Autodesk Fusion 360 part; units mm, degrees
(part 2 of 2)
  arc A307 (-22.8615, 180.477) -> (-23.3615, 180.977) centre (-23.3615, 180.477) ccw
  line L308 (-36.8615, 186.527) -> (-36.8615, 199.527)
  line L309 (-22.8615, 186.527) -> (-22.8615, 199.527)
  line L310 (-36.3615, 186.027) -> (-23.3615, 186.027)
  line L311 (-36.3615, 200.027) -> (-23.3615, 200.027)
  arc A308 (-36.8615, 186.527) -> (-36.3615, 186.027) centre (-36.3615, 186.527) ccw
  arc A309 (-36.3615, 200.027) -> (-36.8615, 199.527) centre (-36.3615, 199.527) ccw
  arc A310 (-23.3615, 186.027) -> (-22.8615, 186.527) centre (-23.3615, 186.527) ccw
  arc A311 (-22.8615, 199.527) -> (-23.3615, 200.027) centre (-23.3615, 199.527) ccw
  line L312 (-36.8615, 205.577) -> (-36.8615, 218.577)
  line L313 (-22.8615, 205.577) -> (-22.8615, 218.577)
  line L314 (-36.3615, 205.077) -> (-23.3615, 205.077)
  line L315 (-36.3615, 219.077) -> (-23.3615, 219.077)
  arc A312 (-36.8615, 205.577) -> (-36.3615, 205.077) centre (-36.3615, 205.577) ccw
  arc A313 (-36.3615, 219.077) -> (-36.8615, 218.577) centre (-36.3615, 218.577) ccw
  arc A314 (-23.3615, 205.077) -> (-22.8615, 205.577) centre (-23.3615, 205.577) ccw
  arc A315 (-22.8615, 218.577) -> (-23.3615, 219.077) centre (-23.3615, 218.577) ccw
  line L316 (-36.8615, 224.627) -> (-36.8615, 237.627)
  line L317 (-22.8615, 224.627) -> (-22.8615, 237.627)
  line L318 (-36.3615, 224.127) -> (-23.3615, 224.127)
  line L319 (-36.3615, 238.127) -> (-23.3615, 238.127)
  arc A316 (-36.8615, 224.627) -> (-36.3615, 224.127) centre (-36.3615, 224.627) ccw
  arc A317 (-36.3615, 238.127) -> (-36.8615, 237.627) centre (-36.3615, 237.627) ccw
  arc A318 (-23.3615, 224.127) -> (-22.8615, 224.627) centre (-23.3615, 224.627) ccw
  arc A319 (-22.8615, 237.627) -> (-23.3615, 238.127) centre (-23.3615, 237.627) ccw
  line L320 (-36.8615, 260.3457) -> (-36.8615, 273.3457)
  line L321 (-22.8615, 260.3457) -> (-22.8615, 273.3457)
  line L322 (-36.3615, 259.8457) -> (-23.3615, 259.8457)
  line L323 (-36.3615, 273.8457) -> (-23.3615, 273.8457)
  arc A320 (-36.8615, 260.3457) -> (-36.3615, 259.8457) centre (-36.3615, 260.3457) ccw
  arc A321 (-36.3615, 273.8457) -> (-36.8615, 273.3457) centre (-36.3615, 273.3457) ccw
  arc A322 (-23.3615, 259.8457) -> (-22.8615, 260.3457) centre (-23.3615, 260.3457) ccw
  arc A323 (-22.8615, 273.3457) -> (-23.3615, 273.8457) centre (-23.3615, 273.3457) ccw
  line L324 (-35.8615, 251.9077) -> (-35.8615, 257.9077)
  line L325 (-20.8615, 251.9077) -> (-20.8615, 257.9077)
  line L326 (-35.3615, 251.4077) -> (-21.3615, 251.4077)
  line L327 (-35.3615, 258.4077) -> (-21.3615, 258.4077)
  arc A324 (-35.8615, 251.9077) -> (-35.3615, 251.4077) centre (-35.3615, 251.9077) ccw
  arc A325 (-35.3615, 258.4077) -> (-35.8615, 257.9077) centre (-35.3615, 257.9077) ccw
  arc A326 (-21.3615, 251.4077) -> (-20.8615, 251.9077) centre (-21.3615, 251.9077) ccw
  arc A327 (-20.8615, 257.9077) -> (-21.3615, 258.4077) centre (-21.3615, 257.9077) ccw
  line L328 (-35.8615, 275.7837) -> (-35.8615, 281.7837)
  line L329 (-20.8615, 275.7837) -> (-20.8615, 281.7837)
  line L330 (-35.3615, 275.2837) -> (-21.3615, 275.2837)
  line L331 (-35.3615, 282.2837) -> (-21.3615, 282.2837)
  arc A328 (-35.8615, 275.7837) -> (-35.3615, 275.2838) centre (-35.3615, 275.7837) ccw
  arc A329 (-35.3615, 282.2837) -> (-35.8615, 281.7837) centre (-35.3615, 281.7837) ccw
  arc A330 (-21.3615, 275.2837) -> (-20.8615, 275.7837) centre (-21.3615, 275.7837) ccw
  arc A331 (-20.8615, 281.7837) -> (-21.3615, 282.2837) centre (-21.3615, 281.7837) ccw
  line L332 (-36.8615, 319.877) -> (-36.8615, 332.877)
  line L333 (-22.8615, 319.877) -> (-22.8615, 332.877)
  line L334 (-36.3615, 319.377) -> (-23.3615, 319.377)
  line L335 (-36.3615, 333.377) -> (-23.3615, 333.377)
  arc A332 (-36.8615, 319.877) -> (-36.3615, 319.377) centre (-36.3615, 319.877) ccw
  arc A333 (-36.3615, 333.377) -> (-36.8615, 332.877) centre (-36.3615, 332.877) ccw
  arc A334 (-23.3615, 319.377) -> (-22.8615, 319.877) centre (-23.3615, 319.877) ccw
  arc A335 (-22.8615, 332.877) -> (-23.3615, 333.377) centre (-23.3615, 332.877) ccw
  line L336 (-17.8115, 12.6957) -> (-17.8115, 25.6957)
  line L337 (-3.8115, 12.6957) -> (-3.8115, 25.6957)
  line L338 (-17.3115, 12.1957) -> (-4.3115, 12.1957)
  line L339 (-17.3115, 26.1957) -> (-4.3115, 26.1957)
  arc A336 (-17.8115, 12.6957) -> (-17.3115, 12.1957) centre (-17.3115, 12.6957) ccw
  arc A337 (-17.3115, 26.1957) -> (-17.8115, 25.6957) centre (-17.3115, 25.6957) ccw
  arc A338 (-4.3115, 12.1957) -> (-3.8115, 12.6957) centre (-4.3115, 12.6957) ccw
  arc A339 (-3.8115, 25.6957) -> (-4.3115, 26.1957) centre (-4.3115, 25.6957) ccw
  line L340 (-17.8115, 36.5082) -> (-17.8115, 49.5082)
  line L341 (-3.8115, 36.5082) -> (-3.8115, 49.5082)
  line L342 (-17.3115, 36.0082) -> (-4.3115, 36.0082)
  line L343 (-17.3115, 50.0082) -> (-4.3115, 50.0082)
  arc A340 (-17.8115, 36.5082) -> (-17.3115, 36.0082) centre (-17.3115, 36.5082) ccw
  arc A341 (-17.3115, 50.0082) -> (-17.8115, 49.5082) centre (-17.3115, 49.5082) ccw
  arc A342 (-4.3115, 36.0082) -> (-3.8115, 36.5082) centre (-4.3115, 36.5082) ccw
  arc A343 (-3.8115, 49.5082) -> (-4.3115, 50.0082) centre (-4.3115, 49.5082) ccw
  line L344 (-17.8115, 60.3207) -> (-17.8115, 73.3207)
  line L345 (-3.8115, 60.3207) -> (-3.8115, 73.3207)
  line L346 (-17.3115, 59.8207) -> (-4.3115, 59.8207)
  line L347 (-17.3115, 73.8207) -> (-4.3115, 73.8207)
  arc A344 (-17.8115, 60.3207) -> (-17.3115, 59.8207) centre (-17.3115, 60.3207) ccw
  arc A345 (-17.3115, 73.8207) -> (-17.8115, 73.3207) centre (-17.3115, 73.3207) ccw
  arc A346 (-4.3115, 59.8207) -> (-3.8115, 60.3207) centre (-4.3115, 60.3207) ccw
  arc A347 (-3.8115, 73.3207) -> (-4.3115, 73.8207) centre (-4.3115, 73.3207) ccw
  line L348 (-17.8115, 131.7582) -> (-17.8115, 144.7582)
  line L349 (-3.8115, 131.7582) -> (-3.8115, 144.7582)
  line L350 (-17.3115, 131.2582) -> (-4.3115, 131.2582)
  line L351 (-17.3115, 145.2582) -> (-4.3115, 145.2582)
  arc A348 (-17.8115, 131.7582) -> (-17.3115, 131.2582) centre (-17.3115, 131.7582) ccw
  arc A349 (-17.3115, 145.2582) -> (-17.8115, 144.7582) centre (-17.3115, 144.7582) ccw
  arc A350 (-4.3115, 131.2582) -> (-3.8115, 131.7582) centre (-4.3115, 131.7582) ccw
  arc A351 (-3.8115, 144.7582) -> (-4.3115, 145.2582) centre (-4.3115, 144.7582) ccw
  line L352 (-16.8115, 85.2582) -> (-16.8115, 91.2582)
  line L353 (-1.8115, 85.2582) -> (-1.8115, 91.2582)
  line L354 (-16.3115, 84.7582) -> (-2.3115, 84.7582)
  line L355 (-16.3115, 91.7582) -> (-2.3115, 91.7582)
  arc A352 (-16.8115, 85.2582) -> (-16.3115, 84.7582) centre (-16.3115, 85.2582) ccw
  arc A353 (-16.3115, 91.7582) -> (-16.8115, 91.2582) centre (-16.3115, 91.2582) ccw
  arc A354 (-2.3115, 84.7582) -> (-1.8115, 85.2582) centre (-2.3115, 85.2582) ccw
  arc A355 (-1.8115, 91.2582) -> (-2.3115, 91.7582) centre (-2.3115, 91.2582) ccw
  line L356 (-16.8115, 185.2582) -> (-16.8115, 191.2582)
  line L357 (-1.8115, 185.2582) -> (-1.8115, 191.2582)
  line L358 (-16.3115, 184.7582) -> (-2.3115, 184.7582)
  line L359 (-16.3115, 191.7582) -> (-2.3115, 191.7582)
  arc A356 (-16.8115, 185.2582) -> (-16.3115, 184.7582) centre (-16.3115, 185.2582) ccw
  arc A357 (-16.3115, 191.7582) -> (-16.8115, 191.2582) centre (-16.3115, 191.2582) ccw
  arc A358 (-2.3115, 184.7582) -> (-1.8115, 185.2582) centre (-2.3115, 185.2582) ccw
  arc A359 (-1.8115, 191.2582) -> (-2.3115, 191.7582) centre (-2.3115, 191.2582) ccw
  line L360 (-17.8115, 203.1958) -> (-17.8115, 216.1957)
  line L361 (-3.8115, 203.1958) -> (-3.8115, 216.1957)
  line L362 (-17.3115, 202.6957) -> (-4.3115, 202.6957)
  line L363 (-17.3115, 216.6957) -> (-4.3115, 216.6957)
  arc A360 (-17.8115, 203.1958) -> (-17.3115, 202.6958) centre (-17.3115, 203.1958) ccw
  arc A361 (-17.3115, 216.6957) -> (-17.8115, 216.1957) centre (-17.3115, 216.1957) ccw
  arc A362 (-4.3115, 202.6957) -> (-3.8115, 203.1958) centre (-4.3115, 203.1958) ccw
  arc A363 (-3.8115, 216.1957) -> (-4.3115, 216.6957) centre (-4.3115, 216.1957) ccw
  line L364 (-17.8115, 227.0082) -> (-17.8115, 240.0082)
  line L365 (-3.8115, 227.0082) -> (-3.8115, 240.0082)
  line L366 (-17.3115, 226.5082) -> (-4.3115, 226.5082)
  line L367 (-17.3115, 240.5082) -> (-4.3115, 240.5082)
  arc A364 (-17.8115, 227.0082) -> (-17.3115, 226.5082) centre (-17.3115, 227.0082) ccw
  arc A365 (-17.3115, 240.5082) -> (-17.8115, 240.0082) centre (-17.3115, 240.0082) ccw
  arc A366 (-4.3115, 226.5082) -> (-3.8115, 227.0082) centre (-4.3115, 227.0082) ccw
  arc A367 (-3.8115, 240.0082) -> (-4.3115, 240.5082) centre (-4.3115, 240.0082) ccw
  line L368 (-17.8115, 250.8207) -> (-17.8115, 263.8207)
  line L369 (-3.8115, 250.8207) -> (-3.8115, 263.8207)
  line L370 (-17.3115, 250.3207) -> (-4.3115, 250.3207)
  line L371 (-17.3115, 264.3207) -> (-4.3115, 264.3207)
  arc A368 (-17.8115, 250.8207) -> (-17.3115, 250.3207) centre (-17.3115, 250.8207) ccw
  arc A369 (-17.3115, 264.3207) -> (-17.8115, 263.8207) centre (-17.3115, 263.8207) ccw
  arc A370 (-4.3115, 250.3207) -> (-3.8115, 250.8207) centre (-4.3115, 250.8207) ccw
  arc A371 (-3.8115, 263.8207) -> (-4.3115, 264.3207) centre (-4.3115, 263.8207) ccw
  line L372 (-17.8115, 274.6332) -> (-17.8115, 287.6332)
  line L373 (-3.8115, 274.6332) -> (-3.8115, 287.6332)
  line L374 (-17.3115, 274.1332) -> (-4.3115, 274.1332)
  line L375 (-17.3115, 288.1332) -> (-4.3115, 288.1332)
  arc A372 (-17.8115, 274.6332) -> (-17.3115, 274.1332) centre (-17.3115, 274.6332) ccw
  arc A373 (-17.3115, 288.1332) -> (-17.8115, 287.6332) centre (-17.3115, 287.6332) ccw
  arc A374 (-4.3115, 274.1332) -> (-3.8115, 274.6332) centre (-4.3115, 274.6332) ccw
  arc A375 (-3.8115, 287.6332) -> (-4.3115, 288.1332) centre (-4.3115, 287.6332) ccw
  line L376 (-17.8115, 300.827) -> (-17.8115, 313.827)
  line L377 (-3.8115, 300.827) -> (-3.8115, 313.827)
  line L378 (-17.3115, 300.327) -> (-4.3115, 300.327)
  line L379 (-17.3115, 314.327) -> (-4.3115, 314.327)
  arc A376 (-17.8115, 300.827) -> (-17.3115, 300.327) centre (-17.3115, 300.827) ccw
  arc A377 (-17.3115, 314.327) -> (-17.8115, 313.827) centre (-17.3115, 313.827) ccw
  arc A378 (-4.3115, 300.327) -> (-3.8115, 300.827) centre (-4.3115, 300.827) ccw
  arc A379 (-3.8115, 313.827) -> (-4.3115, 314.327) centre (-4.3115, 313.827) ccw
  line L380 (-17.8115, 319.877) -> (-17.8115, 332.877)
  line L381 (-3.8115, 319.877) -> (-3.8115, 332.877)
  line L382 (-17.3115, 319.377) -> (-4.3115, 319.377)
  line L383 (-17.3115, 333.377) -> (-4.3115, 333.377)
  arc A380 (-17.8115, 319.877) -> (-17.3115, 319.377) centre (-17.3115, 319.877) ccw
  arc A381 (-17.3115, 333.377) -> (-17.8115, 332.877) centre (-17.3115, 332.877) ccw
  arc A382 (-4.3115, 319.377) -> (-3.8115, 319.877) centre (-4.3115, 319.877) ccw
  arc A383 (-3.8115, 332.877) -> (-4.3115, 333.377) centre (-4.3115, 332.877) ccw
  line L384 (-17.8115, 338.927) -> (-17.8115, 351.927)
  line L385 (-3.8115, 338.927) -> (-3.8115, 351.927)
  line L386 (-17.3115, 338.427) -> (-4.3115, 338.427)
  line L387 (-17.3115, 352.427) -> (-4.3115, 352.427)
  arc A384 (-17.8115, 338.927) -> (-17.3115, 338.427) centre (-17.3115, 338.927) ccw
  arc A385 (-17.3115, 352.427) -> (-17.8115, 351.927) centre (-17.3115, 351.927) ccw
  arc A386 (-4.3115, 338.427) -> (-3.8115, 338.927) centre (-4.3115, 338.927) ccw
  arc A387 (-3.8115, 351.927) -> (-4.3115, 352.427) centre (-4.3115, 351.927) ccw
  circle A388 centre (-48.9265, 345.434) radius 3
  line L388 (-52.4231, 302.396) -> (-42.8615, 302.396)
  line L389 (-42.8615, 302.396) -> (-42.8615, 331.6672)
  line L390 (-42.8615, 331.6672) -> (-52.4231, 331.6672)
  line L391 (-52.4231, 331.6672) -> (-52.4231, 302.396)
  dimension "d76" = 6
  dimension "d77" = 12.057
  dimension "d78" = 12.065
  dimension "d79" = 6
  constraint horizontal L388
  constraint vertical L389
  constraint horizontal L390
  constraint vertical L391
  measures "d76" diameter of A388
  measures "d77" distance of L335 A388.centre
  measures "d78" distance of L332 A388.centre
  measures "d79" distance of L332 L389
sketch "Sketch6" plane through (0, 0, 0) normal (-0.121869, 0, -0.992546) x (0, -1, 0)
  line L0 (0, 24.6165) -> (0, 102.7335)
  line L1 (0, 102.7335) -> (-362.2, 102.7335)
  line L2 (-362.2, 102.7335) -> (-362.2, 24.6165)
  line L3 (-362.2, 24.6165) -> (0, 24.6165)
  line L4 (0, 0) -> (0, -10.166)
  line L5 (0, -10.166) -> (-362.2, -10.166)
  line L6 (-362.2, -10.166) -> (-362.2, 129.834)
  line L7 (-362.2, 129.834) -> (0, 129.834)
  line L8 (0, 129.834) -> (0, 0)
  line L9 (-355.8, 129.834) -> (-355.8, -10.166)
  line L10 (-6.4, 129.834) -> (-6.4, -10.166)
  dimension "d80" = 362.2
  dimension "d81" = 140
  dimension "d82" = 6.4
  dimension "d83" = 6.4
  constraint coincident L4.start L8.end
  constraint vertical L4
  constraint perpendicular L4 L5
  constraint perpendicular L5 L6
  constraint perpendicular L6 L7
  constraint perpendicular L7 L8
  constraint coincident L7 L9.start
  constraint coincident L5 L9.end
  constraint perpendicular L5 L9
  constraint coincident L7 L10.start
  constraint coincident L5 L10.end
  constraint perpendicular L5 L10
  measures "d80" distance of L4.end L5.end
  measures "d81" distance of L5.end L6.end
  measures "d82" distance of L6 L9
  measures "d83" distance of L8 L10
extrude "Extrude2" cut sketch "Sketch6" along normal blind 10 contours L3 L5 L9 L10 | L1 L3 L9 L10 | L1 L7 L9 L10
extrude "Extrude3" cut sketch "plate-2025-12-06T02_04_04.924Z" against normal blind 10
